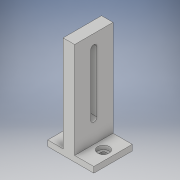
# Autodesk Inventor part: Ventilador tub - guies
Saved by Autodesk Inventor 2019 (Build 230136000, 136)
## iProperties
Created: 2018-08-31
Part Number: Ventilador tub - guies
Material: Genérico
Document SubType Name: Modeling
Designer: Albert Garangou Culebras
Density: 1 g/cm^3
Appearance: Valor por defecto
Author: Albert Garangou Culebras
Autodesk Inventor part; units mm, degrees
ref_plane "YZ Plane" through (0, 0, 0) normal (1, 0, 0) x (0, 1, 0)
ref_plane "XZ Plane" through (0, 0, 0) normal (0, 1, 0) x (-1, 0, 0)
ref_plane "XY Plane" through (0, 0, 0) normal (0, 0, 1) x (1, 0, 0)
sketch "Boceto1" plane through (0, 0, 0) normal (0, 1, 0) x (-1, 0, 0)
  line L0 (0, 0) -> (-10, 0)
  line L1 (-10, -20) -> (0, -20)
  line L2 (-10, 0) -> (-8, 0)
  line L3 (-8, 0) -> (-14, 0)
  line L4 (-14, 0) -> (-18, 0)
  line L5 (-18, 0) -> (-18, -20)
  line L6 (-18, -20) -> (-10, -20)
  line L7 (0, -20) -> (-2, -20)
  line L8 (-2, -20) -> (6, -20)
  line L9 (6, -20) -> (6, 0)
  line L10 (6, 0) -> (0, 0)
  dimension "d8" = 4
  dimension "d9" = 8
  constraints: 22 end point, 5 point on line, 3 perpendicular, 1 horizontal
  measures "d8" distance of L3.end L4.end
  measures "d9" distance of L7.end L8.end
extrude "Extrusión1" add sketch "Boceto1" along normal blind 3
sketch "Boceto2" plane through (0, 3, 0) normal (0, 1, 0) x (1, 0, 0)
  line L0 (5, 20) -> (2, 20)
  line L1 (2, 0) -> (2, 20)
  line L2 (5, 20) -> (8, 20)
  line L3 (8, 0) -> (8, 20)
  line L4 (2, 0) -> (8, 0)
  constraints: 10 end point
extrude "Extrusión2" add sketch "Boceto2" along normal blind 50
sketch "Boceto4" plane through (0, 3, 0) normal (0, 1, 0) x (1, 0, 0)
  line L0 (-6, 0) -> (18, 0) projected
  line L1 (18, 0) -> (8, 0)
  line L2 (13, 0) -> (13, 20)
  point P0 (0, 0)
  point P1 (13, 10)
  constraints: 4 end point, 2 midpoint, 1 point on line, 1 vertical
hole "Agujero2" at (13, 3, -10) direction (0, -1, 0) diameter 3.2 depth 15 counterbore diameter 6 counterbore depth 2
sketch "Boceto5" plane through (0, 3, 0) normal (0, 1, 0) x (1, 0, 0)
  line L0 (-6, 20) -> (-6, 0) projected
  line L1 (-6, 10) -> (2, 10)
  point P0 (0, 0)
  point P1 (-2, 10)
  constraints: 2 end point, 2 midpoint, 1 horizontal
hole "Agujero3" at (-2, 3, -10) direction (0, -1, 0) diameter 3.2 depth 15 counterbore diameter 6 counterbore depth 2
sketch "Boceto6" plane through (8, 3, 0) normal (1, 0, 0) x (0, 0, -1)
  line L0 (10, 10) -> (11.6, 10)
  line L1 (10, 10) -> (8.4, 10)
  line L2 (8.4, 10) -> (8.4, 40)
  line L3 (11.6, 40) -> (11.6, 10)
  line L4 (11.6, 40) -> (11.6, 45)
  line L5 (11.6, 45) -> (8.4, 45)
  line L6 (8.4, 45) -> (8.4, 40)
  point P0 (0, -3)
  constraints: 14 end point, 3 horizontal, 2 perpendicular, 1 vertical
extrude "Extrusión3" cut sketch "Boceto6" against normal blind 35.5
fillet "Empalme1" radius 1.6 4 edges at (5, 48, -11.6) (5, 48, -8.4) (5, 13, -8.4) (5, 13, -11.6)
